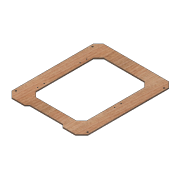
# Autodesk Inventor part: Sides Covers
Saved by Autodesk Inventor 2015 (Build 190159000, 159)
## iProperties
Created: 2018-04-12
Part Number: Sides Covers
Material: Wood (Birch)
Document SubType Name: Modeling
Designer: Ghassan Yusuf
Density: 0.55 g/cm^3
Appearance: Birch - Natural Polished
Author: Ghassan Yusuf
Autodesk Inventor part; units mm, degrees
ref_plane "YZ Plane" through (0, 0, 0) normal (1, 0, 0) x (0, 1, 0)
ref_plane "XZ Plane" through (0, 0, 0) normal (0, 1, 0) x (-1, 0, 0)
ref_plane "XY Plane" through (0, 0, 0) normal (0, 0, 1) x (1, 0, 0)
sketch "Hinges" plane through (0, 0, 0) normal (0, 0, 1) x (1, 0, 0)
  circle A0 centre (-464.8647, 95.9101) radius 1.75
  circle A1 centre (-464.8647, 121.4101) radius 1.75
  line L0 (-471.3647, 88.6601) -> (-455.3647, 88.6601)
  line L1 (-455.3647, 88.6601) -> (-455.3647, 128.6601)
  line L2 (-455.3647, 128.6601) -> (-471.3647, 128.6601)
  line L3 (-471.3647, 128.6601) -> (-471.3647, 88.6601)
  circle A2 centre (-439.8647, 121.4101) radius 1.75
  circle A3 centre (-439.8647, 95.9101) radius 1.75
  line L4 (-433.3647, 128.6601) -> (-449.3647, 128.6601)
  line L5 (-449.3647, 128.6601) -> (-449.3647, 88.6601)
  line L6 (-449.3647, 88.6601) -> (-433.3647, 88.6601)
  line L7 (-433.3647, 88.6601) -> (-433.3647, 128.6601)
  point P0 (-452.3647, 108.6601)
  dimension "d30" = 3.5
  dimension "d31" = 25.5
  dimension "d32" = 6.5
  dimension "d33" = 40
  dimension "d34" = 7.25
  dimension "d35" = 16
  dimension "d36" = 3.5
  dimension "d37" = 25.5
  dimension "d38" = 6.5
  dimension "d39" = 40
  dimension "d40" = 7.25
  dimension "d41" = 16
  dimension "d42" = 38
  measures "d30" diameter of A2
  measures "d31" distance of A3.centre A2.centre
  measures "d32" distance from line of L7 A2.centre
  measures "d33" distance of L6.end L4.start
  measures "d34" distance from line of L6 A3.centre
  measures "d35" distance of L4.start L4.end
  measures "d36" diameter of A0
  measures "d37" distance of A1.centre A0.centre
  measures "d38" distance from line of L3 A0.centre
  measures "d39" distance of L2.end L0.start
  measures "d40" distance from line of L2 A1.centre
  measures "d41" distance of L0.start L0.end
  measures "d42" distance between parallel lines of L7 L3
sketch "Sketch1" plane through (0, 0, 0) normal (0, 0, 1) x (1, 0, 0)
  line L0 (-148.5, 181) -> (148.5, 181)
  line L1 (148.5, 181) -> (148.5, -181)
  line L2 (148.5, -181) -> (-148.5, -181)
  line L3 (-148.5, -181) -> (-148.5, 181)
  line L4 (-75, -181) -> (-65, -171)
  line L5 (-75, -181) -> (-60.8579, -181) construction
  line L6 (-65, -171) -> (65, -171)
  line L7 (65, -171) -> (75, -181)
  line L8 (-125, -181) -> (-148.5, -157.5)
  line L9 (-125, -181) -> (-91.766, -181) construction
  line L10 (125, -181) -> (148.5, -157.5)
  line L11 (125, -181) -> (158.234, -181) construction
  line L12 (-148.5, 161) -> (-128.5, 181)
  line L13 (-148.5, 161) -> (-120.2157, 161) construction
  line L14 (148.5, 161) -> (128.5, 181)
  line L15 (-100, 134) -> (100, 134)
  line L16 (100, 134) -> (100, -133)
  line L17 (100, -133) -> (-100, -133)
  line L18 (-100, -133) -> (-100, 134)
  point P0 (0, 0)
  point P1 (0, 181)
  point P2 (-148.5, 0)
  point P3 (0, -171)
  point P4 (0, 134)
  dimension "d0" = 297
  dimension "d1" = 362
  dimension "d2" = 45
  dimension "d3" = 10
  dimension "d4" = 150
  dimension "d5" = 135
  dimension "d6" = 50
  dimension "d7" = 45
  dimension "d8" = 50
  dimension "d9" = 45
  dimension "d10" = 20
  dimension "d11" = 20
  dimension "d12" = 135
  dimension "d13" = 47
  dimension "d14" = 200
  dimension "d15" = 267
  constraints: 38 end point, 10 point on line, 7 horizontal, 5 equal length, 4 midpoint, 4 parallel, 3 perpendicular, 3 vertical alignment, 1 horizontal alignment
  measures "d0" distance of L1.end L2.end
  measures "d1" distance of L0.end L1.end
  measures "d2" angle of L5 L4
  measures "d3" distance between parallel lines of L2 L6
  measures "d4" distance of L7.end L4.start
  measures "d5" angle of L9 L8
  measures "d6" distance of L4.start L8.start
  measures "d7" angle of L11 L10
  measures "d8" distance of L10.start L7.end
  measures "d9" angle of L13 L12
  measures "d10" distance of L0.start L12.start
  measures "d11" distance of L0.end L14.start
  measures "d12" angle of L14 L1
  measures "d13" distance between parallel lines of L0 L15
  measures "d14" distance of L16.end L17.end
  measures "d15" distance between parallel lines of L17 L15
extrude "Extrusion1" add sketch "Sketch1" along normal mid plane 4 contours L0 L14 L1 L10 L2 L7 L6 L4 L8 L3 L12
chamfer "Chamfer1" distance 20 angle 45 4 edges at (-100, 134, 0) (100, 134, 0) (-100, -133, 0) (100, -133, 0)
sketch "Sketch3" plane through (0, 0, -2) normal (0, 0, -1) x (-1, 0, 0)
  circle A0 centre (-140.5, 150) radius 3
  circle A1 centre (-140.5, -150) radius 3
  circle A2 centre (140.5, -150) radius 3
  circle A3 centre (140.5, 150) radius 3
  line L0 (-148.5, 161) -> (-148.5, -157.5) projected
  line L1 (148.5, -157.5) -> (148.5, 161) projected
  point P0 (0, 0)
  dimension "d25" = 6
  dimension "d26" = 300
  dimension "d27" = 150
  dimension "d47" = 8
  dimension "d48" = 8
  constraints: 4 centre point, 3 equal radius, 2 horizontal alignment, 2 vertical alignment
  measures "d25" diameter of A0
  measures "d26" distance of A1.centre A0.centre
  measures "d27" vertical distance of point (0, 0) A0.centre
  measures "d47" distance from line of L0 A0.centre
  measures "d48" distance from line of L1 A3.centre
extrude "Extrusion3" cut sketch "Sketch3" against normal blind 37.5
sketch "Sketch4" plane through (0, 0, -2) normal (0, 0, -1) x (-1, 0, 0)
  line L0 (100, 114) -> (100, -113) projected
  line L1 (-100, -113) -> (-100, 114) projected
  circle A0 centre (84.5, 71.25) radius 1.75
  circle A1 centre (84.5, 96.75) radius 1.75
  line L2 (78, 64) -> (94, 64)
  line L3 (94, 64) -> (94, 104)
  line L4 (94, 104) -> (78, 104)
  line L5 (78, 104) -> (78, 64)
  circle A2 centre (109.5, 96.75) radius 1.75
  circle A3 centre (109.5, 71.25) radius 1.75
  line L6 (116, 104) -> (100, 104)
  line L7 (100, 104) -> (100, 64)
  line L8 (100, 64) -> (116, 64)
  line L9 (116, 64) -> (116, 104)
  circle A4 centre (84.5, -95.75) radius 1.75
  circle A5 centre (84.5, -70.25) radius 1.75
  line L10 (78, -103) -> (94, -103)
  line L11 (94, -103) -> (94, -63)
  line L12 (94, -63) -> (78, -63)
  line L13 (78, -63) -> (78, -103)
  circle A6 centre (109.5, -70.25) radius 1.75
  circle A7 centre (109.5, -95.75) radius 1.75
  line L14 (116, -63) -> (100, -63)
  line L15 (100, -63) -> (100, -103)
  line L16 (100, -103) -> (116, -103)
  line L17 (116, -103) -> (116, -63)
  circle A8 centre (-109.5, -12.75) radius 1.75
  circle A9 centre (-109.5, 12.75) radius 1.75
  line L18 (-116, -20) -> (-100, -20)
  line L19 (-100, -20) -> (-100, 20)
  line L20 (-100, 20) -> (-116, 20)
  line L21 (-116, 20) -> (-116, -20)
  circle A10 centre (-84.5, 12.75) radius 1.75
  circle A11 centre (-84.5, -12.75) radius 1.75
  line L22 (-78, 20) -> (-94, 20)
  line L23 (-94, 20) -> (-94, -20)
  line L24 (-94, -20) -> (-78, -20)
  line L25 (-78, -20) -> (-78, 20)
  point P0 (0, 0)
  point P1 (-100, 0)
  dimension "d43" = 10
  dimension "d44" = 10
  constraints: 3 vertical, 1 horizontal alignment, 1 other
extrude "Extrusion4" cut sketch "Sketch4" against normal blind 10 contours A2 | A3 | A6 | A7 | A8 | A9
equation "\"d27\" = 0.5 * d26"
equation "\"d34\" = -0.5 * d31 + 0.5 * d33"
equation "\"d40\" = -0.5 * d37 + 0.5 * d39"
equation "\"d8\" = d6"
equation "\"d48\" = d47"
body "Solid1"
